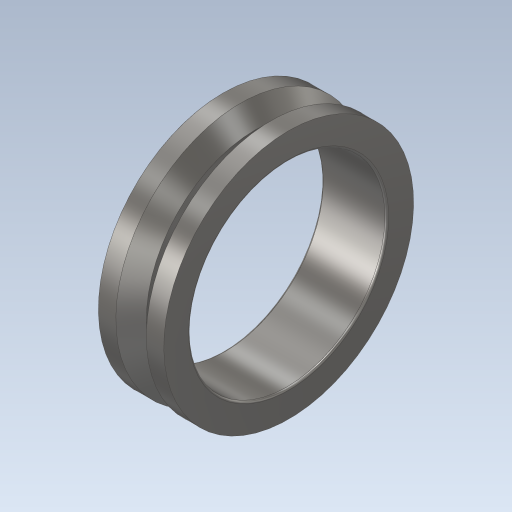
# Autodesk Inventor part: CRBT155A_PART1
Saved by Autodesk Inventor 2024 (Build 280153000, 153)
## iProperties
Created: 2023-09-04
Part Number: CRBT155A_PART1
Material: ステンレス鋼
Catalog Web Link: www.cadenas.de
Description: -
Vendor: IKO
Document SubType Name: Modeling
Designer: psAdmin
Manufacturer: IKO
Mass: 3.76441 g
Surface Area: 7.95035 cm^2
Volume: 0.470551 cm^3
Density: 8 g/cm^3
Appearance: 半つや出し
Category: PARTsolutions
Company: IKO
PSOL_IDENT_0: {$CADENAS_DATA/23d-libs/iko/iko_bearings/crossed_rb/ultra_slim_type_crb/ultra_slim_type_crbt.prj},23
PSOL_IDENT_1: 2 {VTYP=3D},{NB=CRBT155A_PART1},{LINA=CRBT155A_PART1},{NN=Ultra Slim Type Crossed Roller Bearings (C
PSOL_IDENT_2: RBT...A)_PART1},{NOPRJ=TRUE},{DATE=09.07.2020 23:28:49},{GEOMDATE=08.07.2020 06:24:28},{VERSION=},{L
PSOL_IDENT_3: INEID=220},{WBVAR=},{WBNUMERIC=}  {NB=CRBT155A_PART1},{LINA=CRBT155A_PART1},{KT=DUMMY},{IDNR=},{STDR
PSOL_IDENT_4: T=15},{ORDER=CRBT155A},{MASS=11.9},{SD=15},{D=26},{B=5},{SR=0.15},{SDA=17.5},{DA=22.0},{DAR=2.0},{ZE
PSOL_IDENT_5: FF=16},{RS=0.3},{DETC=1.6},{PCDRL=19.6},{SDOR=20.10},{DIRR=19.10},{COG=0.0},{SDOG=0.0},{OH=0.0},{NH=
PSOL_IDENT_6: 0},{CR=1320},{COR=1110},{SC=0},{N=8},{N1=1.67}
NB: CRBT155A_PART1
NBSYN: $ORDER._PART1
LINA: CRBT155A_PART1
CATALOG: IKO (Nippon Thompson
STDRT: 15
ORDER: CRBT155A
MASS: 11.9
SD: 15
D: 26
B: 5
SR: 0.15
SDA: 17.5
DA: 22
CR: 1320
COR: 1110
SUPPLIER: IKO
ARTICLENO: CRBT155A_PART1
BOMINFO: CRBT155A_PART1
CREATOR: CADENAS GmbH
Title: CRBT155A_PART1
Author: Cadenas PARTsolutions
Autodesk Inventor part; units mm, degrees
ref_plane "YZ Plane" through (0, 0, 0) normal (1, 0, 0) x (0, 1, 0)
ref_plane "XZ Plane" through (0, 0, 0) normal (0, 1, 0) x (-1, 0, 0)
ref_plane "XY Plane" through (0, 0, 0) normal (0, 0, 1) x (1, 0, 0)
sketch "Sketch_1" plane through (0, 0, 0) normal (0, 0, 1) x (1, 0, 0)
  line L0 (5, 0) -> (0, 0)
  arc A0 (0, 7.65) -> (0.15, 7.5) centre (0.15, 7.65) ccw
  line L1 (0.15, 7.5) -> (4.85, 7.5)
  arc A1 (4.85, 7.5) -> (5, 7.65) centre (4.85, 7.65) ccw
  line L2 (5, 7.65) -> (5, 9.55)
  line L3 (5, 9.55) -> (0, 9.55)
  line L4 (0, 9.55) -> (0, 7.65)
  constraints: 10 end point, 4 point on circle, 2 centre point
revolve "Revolution1" add sketch "Sketch_1" angle 360 about axis through (5, 0, 0) along (1, 0, 0)
sketch "Sketch_2" plane through (0, 0, 0) normal (0, 0, 1) x (1, 0, 0)
  line L0 (3.5, 0) -> (1.5, 0)
  line L1 (1.0858, 9.8) -> (2.5, 8.3858)
  line L2 (2.5, 8.3858) -> (3.9142, 9.8)
  line L3 (3.9142, 9.8) -> (2.5, 11.2142)
  line L4 (2.5, 11.2142) -> (1.0858, 9.8)
  constraints: 10 end point
revolve "Revolution2" cut sketch "Sketch_2" angle 360 about axis through (3.5, 0, 0) along (1, 0, 0)
body "Solid1"
